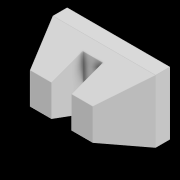
# Autodesk Inventor part: 零件3
Saved by Autodesk Inventor 2020 (Build 240168000, 168)
## iProperties
Created: 2020-11-12
Part Number: 零件3
Material: 常规
Document SubType Name: Modeling
Designer: NH55
Density: 1 g/cm^3
Appearance: 默认
Author: NH55
Autodesk Inventor part; units mm, degrees
ref_plane "YZ Plane" through (0, 0, 0) normal (1, 0, 0) x (0, 1, 0)
ref_plane "XZ Plane" through (0, 0, 0) normal (0, 1, 0) x (-1, 0, 0)
ref_plane "XY Plane" through (0, 0, 0) normal (0, 0, 1) x (1, 0, 0)
sketch "草图2" plane through (0, 0, 0) normal (0, 1, 0) x (-1, 0, 0)
  line L0 (-18, 0) -> (18, 0)
  line L1 (18, 0) -> (18, 5)
  line L2 (18, 5) -> (-18, 5)
  line L3 (-18, 5) -> (-18, 0)
  line L4 (-18, 5) -> (-11, 20)
  line L5 (-11, 20) -> (-3.5, 20)
  line L6 (-3.5, 20) -> (-3.5, 9)
  line L7 (-3.5, 9) -> (3.5, 9)
  line L8 (3.5, 9) -> (3.5, 20)
  line L9 (3.5, 20) -> (11, 20)
  line L10 (11, 20) -> (18, 5)
  point P0 (0, 0)
  point P1 (0, 0)
  point P2 (0, 5)
  point P3 (0, 9)
  dimension "d0" = 36
  dimension "d1" = 5
  dimension "d2" = 20
  dimension "d3" = 11
  dimension "d4" = 7
  dimension "d5" = 22
  constraints: 22 end point, 7 perpendicular, 3 midpoint, 2 coincident, 2 point on line, 2 vertical alignment, 1 equal length, 1 horizontal
  measures "d0" distance of L0.start L0.end
  measures "d1" distance of L2.end L0.start
  measures "d2" distance between parallel lines of L0 L5
  measures "d3" distance between parallel lines of L9 L7
  measures "d4" distance of L6.end L7.end
  measures "d5" distance of L4.end L9.end
extrude "拉伸1" add sketch "草图2" along normal mid plane 22 contours L3 L2 L1 L0
extrude "拉伸2" add sketch "草图2" along normal mid plane 22 contours L4 L5 L6 L7 L8 L9 L10 L2
sketch "草图3" plane through (18, -11, 0) normal (1, 0, 0) x (0, 0, -1)
  line L0 (-5, 22) -> (-5, 0) projected
  line L1 (-20, 22) -> (-5, 22) projected
  line L2 (-20, 0) -> (-20, 22) projected
  line L3 (-5, 0) -> (-20, 0) projected
  line L4 (0, 0) -> (0, 22) projected
  line L5 (-5, 22) -> (0, 22) projected
  line L6 (-5, 22) -> (-5, 0) projected
  line L7 (0, 0) -> (-5, 0) projected
  line L8 (-5, 0) -> (-20, 5.5)
  line L9 (-5, 22) -> (-20, 16.5)
  line L10 (-20, 0) -> (-20, 22) projected
  line L11 (-20, 16.5) -> (-20, 5.5)
  line L12 (-5, 0) -> (-5, 22) projected
  line L13 (-5, 0) -> (-5, 22)
  line L14 (-5, 0) -> (0, 0)
  line L15 (0, 0) -> (0, 22) projected
  line L16 (0, 22) -> (0, 0)
  line L17 (-5, 22) -> (0, 22) projected
  line L18 (-5, 22) -> (0, 22)
  point P0 (0, 11)
  dimension "d10" = 11
  constraints: 14 end point, 2 collinear, 2 point on line, 2 vertical, 1 equal length, 1 horizontal
  measures "d10" distance of L9.end L8.end
extrude "拉伸3" cut sketch "草图3" against normal blind 36 contours L5 L4 L7 L0 | L0 L8 L2 L9 keep common part
